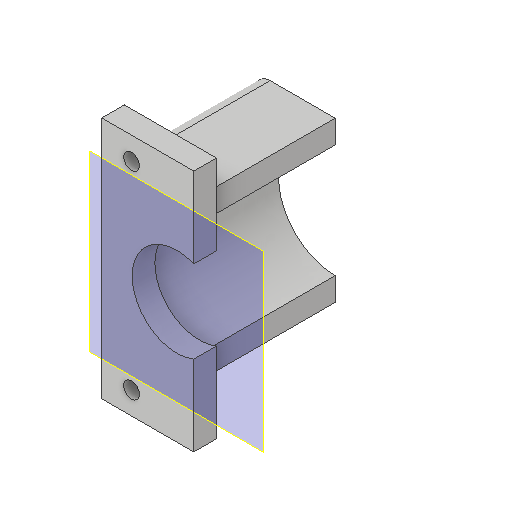
# Autodesk Inventor part: 30_Cube_Z_Focus_MGN_NEMA_Motoradapter_NEMA11_v3
Saved by Autodesk Inventor 2022 (Build 260153000, 153)
## iProperties
Created: 2021-10-20
Part Number: 30_Cube_Z_Focus_MGN_NEMA_Motoradapter_NEMA11_v3
Material: Generic
Document SubType Name: Modeling
Designer: diederichbenedict
Density: 1 g/cm^3
Appearance: Default
Author: diederichbenedict
Autodesk Inventor part; units mm, degrees
ref_plane "YZ Plane" through (0, 0, 0) normal (1, 0, 0) x (0, 1, 0)
ref_plane "XZ Plane" through (0, 0, 0) normal (0, 1, 0) x (-1, 0, 0)
ref_plane "Work Plane3" through (-9.83, 0, 22) normal (0, 0, -1) x (0, -1, 0)
sketch "Sketch2" plane through (-9.83, 0, 22) normal (0, 0, -1) x (0, -1, 0)
  arc A0 (-15.4, 8) -> (-19.6, 8) centre (-17.5, 8) ccw projected
  circle A1 centre (17.5, 8) radius 2.1 projected
  circle A2 centre (-17.5, 8) radius 1.4
  circle A3 centre (17.5, 8) radius 1.4
  arc A4 (-11.5, 14) -> (-14, 11.5) centre (-11.5, 11.5) ccw construction
  arc A5 (14, 11.5) -> (11.5, 14) centre (11.5, 11.5) ccw construction
  line L0 (-21.5, 13.2678) -> (21.5, 13.2678)
  line L1 (21.5, 13.2678) -> (21.5, -3)
  line L2 (-21.5, -3) -> (-21.5, 13.2678)
  arc A6 (-2.1271, -1.5804) -> (-2.4402, 1.0334) centre (0, 0) ccw projected
  arc A7 (7.2826, -3) -> (-7.2826, -3) centre (0, 0) ccw
  line L3 (21.5, -3) -> (7.2826, -3)
  line L4 (-7.2826, -3) -> (-21.5, -3)
  dimension "d26" = 2.8
  dimension "d27" = 2.8
  dimension "d28" = 4
  dimension "d29" = 4
  constraints: 10 end point, 3 centre point, 3 coincident, 3 parallel, 2 point on circle, 1 horizontal, 1 perpendicular
  measures "d26" diameter of A2
  measures "d27" diameter of A3
  measures "d28" distance from line of L2 A0.centre
  measures "d29" distance from line of L1 A1.centre
extrude "Extrusion2" add sketch "Sketch2" along normal blind 4 contours A1 | L0 L1 L3 A7 L4 L2
sketch "Sketch3" plane through (-9.83, 0, 18) normal (0, 0, -1) x (-1, 0, 0)
  circle A0 centre (0, 0) radius 12.75 projected
  circle A1 centre (11.5, 11.5) radius 1.025 projected
  circle A2 centre (11.5, -11.5) radius 1.025 projected
  circle A3 centre (-11.5, -11.5) radius 1.025 projected
  circle A4 centre (-11.5, 11.5) radius 1.025 projected
  line L0 (-11.5, -14.1) -> (11.5, -14.1) projected
  arc A5 (11.5, -14.1) -> (14.1, -11.5) centre (11.5, -11.5) ccw projected
  line L1 (14.1, -11.5) -> (14.1, 11.5) projected
  arc A6 (14.1, 11.5) -> (11.5, 14.1) centre (11.5, 11.5) ccw projected
  line L2 (11.5, 14.1) -> (-11.5, 14.1) projected
  arc A7 (-11.5, 14.1) -> (-14.1, 11.5) centre (-11.5, 11.5) ccw projected
  line L3 (-14.1, 11.5) -> (-14.1, -11.5) projected
  arc A8 (-14.1, -11.5) -> (-11.5, -14.1) centre (-11.5, -11.5) ccw projected
  line L4 (-11.5, -14.1) -> (11.5, -14.1) projected
  line L5 (0, -14.1) -> (0, -12.75)
  line L6 (0, 12.75) -> (0, 14.1)
  line L7 (11.5, 14.1) -> (-11.5, 14.1) projected
  circle A9 centre (0, 0) radius 10
  line L8 (0, -10) -> (0, -12.75)
  line L9 (0, 10) -> (0, 12.75)
  point P0 (-9.83, 0)
  dimension "d11" = 20
  constraints: 8 end point, 4 point on circle, 2 collinear, 2 midpoint, 2 point on line, 1 centre point, 1 coincident, 1 perpendicular
  measures "d11" diameter of A9
ref_plane "Work Plane4" through (-37.83, -24.85, 0) normal (0, 0, -1) x (0, 1, 0)
extrude "Extrusion3" add sketch "Sketch3" along normal blind 24 contours A0 L8 A9 L9 | A0 L6 L2 A6 L1 A5 L0 L5 picked at (11.7268, -0.9457)
sketch "Sketch4" plane through (-9.83, -14.1, -6) normal (0, 0, -1) x (-1, 0, 0)
  circle A0 centre (4.2632, 2.351) radius 1.4
  circle A1 centre (11.5541, 7.5847) radius 1.4
  arc A2 (0, 4.1) -> (0, 24.1) centre (0, 14.1) ccw projected
  line L0 (10, 14.1) -> (14.0989, 14.1)
  circle A3 centre (4.2632, 25.849) radius 1.4
  circle A4 centre (11.5541, 20.6153) radius 1.4
  point P0 (-9.83, 14.1)
  dimension "d16" = 2.8
  dimension "d17" = 2.8
  constraints: 4 centre point, 2 end point, 2 symmetric about line, 1 horizontal, 1 point on circle, 2 other
  measures "d16" diameter of A0
  measures "d17" diameter of A1
extrude "Extrusion4" cut sketch "Sketch4" against normal blind 15
body "Solid2"
